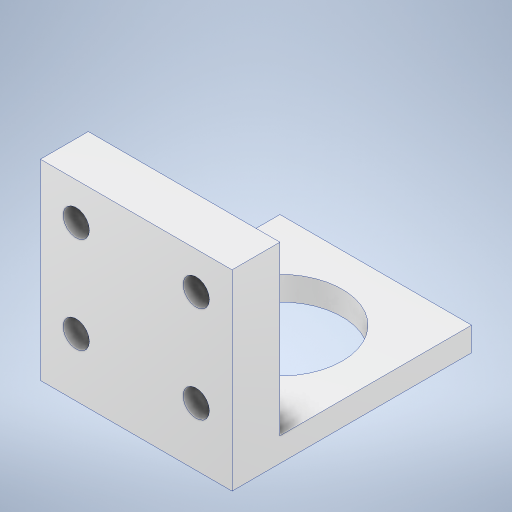
# Autodesk Inventor part: Suporte da guia do eixo
Saved by Autodesk Inventor 2023 (Build 270158000, 158)
## iProperties
Created: 2023-03-22
Part Number: Suporte da guia do eixo
Material: Alumínio 6061
Document SubType Name: Sheet Metal
Designer: Mateus PC
Density: 2.7 g/cm^3
Sheet Metal Rule: Default_mm
Appearance: Alumínio - Plano
Author: Mateus
Autodesk Inventor part; units mm, degrees
ref_plane "YZ Plane" through (0, 0, 0) normal (1, 0, 0) x (0, 1, 0)
ref_plane "XZ Plane" through (0, 0, 0) normal (0, 1, 0) x (-1, 0, 0)
ref_plane "XY Plane" through (0, 0, 0) normal (0, 0, 1) x (1, 0, 0)
sketch "Esboço1" plane through (0, 0, 0) normal (0, 1, 0) x (-1, 0, 0)
  line L0 (0, 0) -> (40, 0)
  line L1 (40, 0) -> (40, -50)
  line L2 (40, -50) -> (0, -50)
  line L3 (0, -50) -> (0, 0)
  dimension "d0" = 40
  dimension "d1" = 50
  constraints: 8 end point, 2 parallel, 1 horizontal, 1 perpendicular
  measures "d0" distance of L1.end L2.end
  measures "d1" distance of L0.end L1.end
extrude "Extrusão1" add sketch "Esboço1" along normal blind 5
sketch "Esboço2" plane through (0, 5, 0) normal (0, 1, 0) x (1, 0, 0)
  line L0 (-40, 50) -> (-40, 0) projected
  line L1 (0, 0) -> (-40, 0)
  line L2 (-40, 0) -> (-40, 10)
  line L3 (-40, 10) -> (0, 10)
  line L4 (0, 10) -> (0, 0)
  point P0 (-40, 0)
  dimension "d4" = 10
  constraints: 8 end point, 2 parallel, 1 horizontal, 1 perpendicular, 1 point on line
  measures "d4" distance between parallel lines of L1 L3
extrude "Extrusão2" add sketch "Esboço2" along normal blind 35
sketch "Esboço3" plane through (0, 5, 0) normal (0, 1, 0) x (1, 0, 0)
  line L0 (-40, 50) -> (-40, 10) projected
  line L1 (0, 50) -> (-40, 50) projected
  point P0 (0, 0)
  point P1 (-20, 30)
  dimension "d7" = 40
  dimension "d8" = 40
  dimension "d9" = 20
  dimension "d10" = 20
  measures "d7" distance of L0.start L0.end
  measures "d8" distance of L1.start L0.start
  measures "d9" distance from line of L0 point (-20, 30)
  measures "d10" distance from line of L1 point (-20, 30)
hole "Furo1" at (-20, 5, -30) direction (0, -1, 0) diameter 26 end through all
sketch "Sketch4" plane through (-40, 0, 0) normal (0, 0, 1) x (1, 0, 0)
  line L0 (0, 0) -> (0, 40) projected
  line L1 (0, 40) -> (40, 40) projected
  point P0 (40, 0)
  point P1 (7.475, 12.15)
  point P2 (7.475, 32.25)
  point P3 (32.525, 12.15)
  point P4 (32.525, 32.25)
  dimension "d20" = 20.1
  dimension "d23" = 25.05
  dimension "d26" = 7.75
  dimension "d27" = 40
  dimension "d28" = 7.475
  constraints: 1 horizontal, 1 vertical, 3 other
  measures "d20" distance of point (7.475, 12.15) point (7.475, 32.25)
  measures "d23" distance of point (7.475, 12.15) point (32.525, 12.15)
  measures "d26" distance from line of L1 point (7.475, 32.25)
  measures "d27" distance of L0.end L1.end
  measures "d28" distance from line of L0 point (7.475, 32.25)
hole "Hole2" at (-32.525, 12.15, 0) at (-32.525, 32.25, 0) at (-7.475, 12.15, 0) at (-7.475, 32.25, 0) direction (0, 0, -1) diameter 5.5 end through all
equation "\"d9\" = 0.5 * d8"
equation "\"d10\" = 0.5 * d7"
equation "\"d16\" = Espessura"
equation "\"d28\" = -0.5 * d23 + 0.5 * d27"
equation "\"d34\" = Espessura"
equation "\"Raio_vergadura\" = Espessura"
equation "\"Largura_alívio_de_vergadura\" = Espessura"
equation "\"Profundidade_alívio_de_vergadura\" = 0.5 * Espessura"
equation "\"Tamanho_alívio_de_dobra\" = 4 * Espessura"
equation "\"Remanescente_mínimo\" = 2 * Espessura"
equation "\"Raiodetransição\" = Raio_vergadura"
equation "\"Tamanho_de_raio_de_Jacobi\" = Raio_vergadura"
equation "\"TamanhoFolga\" = Espessura"
equation "\"Espessura\" = 0.5"
